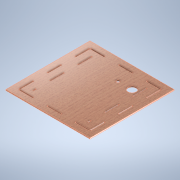
# Autodesk Inventor part: Roof_V2
Saved by Autodesk Inventor 2022.2 (Build 262287000, 287)
## iProperties
Created: 2022-11-15
Part Number: Roof_V2
Material: Generic
Document SubType Name: Modeling
Designer: jaege
Density: 1 g/cm^3
Appearance: Red Oak - Natural Low Gloss
Mass: 344.053 g
Surface Area: 1843.39 cm^2
Volume: 344.053 cm^3
Author: jaege
Autodesk Inventor part; units mm, degrees
ref_plane "YZ Plane" through (0, 0, 0) normal (1, 0, 0) x (0, 1, 0)
ref_plane "XZ Plane" through (0, 0, 0) normal (0, 1, 0) x (-1, 0, 0)
ref_plane "XY Plane" through (0, 0, 0) normal (0, 0, 1) x (1, 0, 0)
sketch "Sketch1" plane through (0, 0, 0) normal (0, 0, 1) x (1, 0, 0)
  line L0 (120, -66) -> (20, -66) construction
  line L1 (20, -66) -> (20, -26) construction
  line L2 (20, -26) -> (120, -26) construction
  line L3 (120, -26) -> (120, -66) construction
  line L4 (-275, -71) -> (125, -71) construction
  line L5 (125, -71) -> (125, 329) construction
  line L6 (125, 329) -> (-275, 329) construction
  line L7 (-275, 329) -> (-275, -71) construction
  line L8 (50, 104) -> (50, 154) construction
  line L9 (50, 154) -> (54, 154) construction
  line L10 (54, 154) -> (54, 104) construction
  line L11 (54, 104) -> (50, 104) construction
  line L12 (-50, 254) -> (-100, 254) construction
  line L13 (-100, 254) -> (-100, 258) construction
  line L14 (-100, 258) -> (-50, 258) construction
  line L15 (-50, 258) -> (-50, 254) construction
  line L16 (50, 258) -> (50, 254) construction
  line L17 (50, 254) -> (54, 254) construction
  line L18 (54, 254) -> (54, 204) construction
  line L19 (54, 204) -> (50, 204) construction
  line L20 (50, 204) -> (50, 254) construction
  line L21 (50, 254) -> (0, 254) construction
  line L22 (0, 254) -> (0, 258) construction
  line L23 (0, 258) -> (50, 258) construction
  line L24 (54, 4) -> (50, 4) construction
  line L25 (50, 4) -> (50, 0) construction
  line L26 (50, 0) -> (0, 0) construction
  line L27 (0, 0) -> (0, 4) construction
  line L28 (0, 4) -> (50, 4) construction
  line L29 (50, 4) -> (50, 54) construction
  line L30 (50, 54) -> (54, 54) construction
  line L31 (54, 54) -> (54, 4) construction
  line L32 (-100, 4) -> (-50, 4) construction
  line L33 (-50, 4) -> (-50, 0) construction
  line L34 (-50, 0) -> (-100, 0) construction
  line L35 (-100, 0) -> (-100, 4) construction
  line L36 (-204, 254) -> (-200, 254) construction
  line L37 (-200, 254) -> (-200, 258) construction
  line L38 (-200, 258) -> (-150, 258) construction
  line L39 (-150, 258) -> (-150, 254) construction
  line L40 (-150, 254) -> (-200, 254) construction
  line L41 (-200, 254) -> (-200, 204) construction
  line L42 (-200, 204) -> (-204, 204) construction
  line L43 (-204, 204) -> (-204, 254) construction
  line L44 (-200, 154) -> (-200, 104) construction
  line L45 (-200, 104) -> (-204, 104) construction
  line L46 (-204, 104) -> (-204, 154) construction
  line L47 (-204, 154) -> (-200, 154) construction
  line L48 (-200, 54) -> (-200, 4) construction
  line L49 (-200, 4) -> (-150, 4) construction
  line L50 (-150, 4) -> (-150, 0) construction
  line L51 (-150, 0) -> (-200, 0) construction
  line L52 (-200, 0) -> (-200, 4) construction
  line L53 (-200, 4) -> (-204, 4) construction
  line L54 (-204, 4) -> (-204, 54) construction
  line L55 (-204, 54) -> (-200, 54) construction
  line L56 (-275, -71) -> (125, -71) construction
  line L57 (125, -71) -> (125, 329) construction
  line L58 (125, 329) -> (-275, 329) construction
  line L59 (-275, 329) -> (-275, -71) construction
  line L60 (-275, -71) -> (125, 329) construction
  line L61 (75, 279) -> (-225, 279)
  line L62 (-225, 279) -> (-225, -21)
  line L63 (-225, -21) -> (75, -21)
  line L64 (75, -21) -> (75, 279)
  line L65 (75, 279) -> (-225, -21) construction
  line L66 (-225, 279) -> (75, -21) construction
  line L67 (-204, 4) -> (-200, 4)
  line L68 (-200, 4) -> (-200, 54)
  line L69 (-200, 54) -> (-204, 54)
  line L70 (-204, 54) -> (-204, 4)
  line L71 (-200, 104) -> (-204, 104)
  line L72 (-204, 104) -> (-204, 154)
  line L73 (-204, 154) -> (-200, 154)
  line L74 (-200, 154) -> (-200, 104)
  line L75 (-200, 204) -> (-204, 204)
  line L76 (-204, 204) -> (-204, 254)
  line L77 (-204, 254) -> (-200, 254)
  line L78 (-200, 254) -> (-200, 204)
  line L79 (-200, 254) -> (-150, 254)
  line L80 (-150, 254) -> (-150, 258)
  line L81 (-150, 258) -> (-200, 258)
  line L82 (-200, 258) -> (-200, 254)
  line L83 (-100, 254) -> (-50, 254)
  line L84 (-50, 254) -> (-50, 258)
  line L85 (-50, 258) -> (-100, 258)
  line L86 (-100, 258) -> (-100, 254)
  line L87 (0, 254) -> (50, 254)
  line L88 (50, 254) -> (50, 258)
  line L89 (50, 258) -> (0, 258)
  line L90 (0, 258) -> (0, 254)
  line L91 (50, 254) -> (54, 254)
  line L92 (54, 254) -> (54, 204)
  line L93 (54, 204) -> (50, 204)
  line L94 (50, 204) -> (50, 254)
  line L95 (54, 154) -> (50, 154)
  line L96 (50, 154) -> (50, 104)
  line L97 (50, 104) -> (54, 104)
  line L98 (54, 104) -> (54, 154)
  line L99 (54, 4) -> (50, 4)
  line L100 (50, 4) -> (50, 54)
  line L101 (50, 54) -> (54, 54)
  line L102 (54, 54) -> (54, 4)
  line L103 (50, 4) -> (0, 4)
  line L104 (0, 4) -> (0, 0)
  line L105 (0, 0) -> (50, 0)
  line L106 (50, 0) -> (50, 4)
  line L107 (-100, 0) -> (-50, 0)
  line L108 (-50, 0) -> (-50, 4)
  line L109 (-50, 4) -> (-100, 4)
  line L110 (-100, 4) -> (-100, 0)
  line L111 (-200, 0) -> (-150, 0)
  line L112 (-150, 0) -> (-150, 4)
  line L113 (-150, 4) -> (-200, 4)
  line L114 (-200, 4) -> (-200, 0)
  point P0 (-75, 129)
  dimension "d0" = 300
  dimension "d1" = 300
  constraints: 118 end point, 28 parallel, 14 horizontal, 14 perpendicular, 3 midpoint
  measures "d0" distance of L63.end L62.end
  measures "d1" distance of L62.end L61.end
extrude "Extrusion1" add sketch "Sketch1" against normal blind 4
sketch "Sketch2" plane through (0, 0, 0) normal (0, 0, 1) x (1, 0, 0)
  line L0 (-175, 234) -> (-171, 234)
  line L1 (-171, 234) -> (-171, 184)
  line L2 (-171, 184) -> (-175, 184)
  line L3 (-175, 184) -> (-175, 234)
  line L4 (-175, 184) -> (-171, 184)
  line L5 (-171, 184) -> (-171, 134)
  line L6 (-171, 134) -> (-175, 134)
  line L7 (-175, 134) -> (-175, 184)
  line L8 (-175, 134) -> (-171, 134)
  line L9 (-171, 134) -> (-171, 84)
  line L10 (-171, 84) -> (-175, 84)
  line L11 (-175, 84) -> (-175, 134)
  line L12 (-200, 254) -> (-200, 204) projected
  line L13 (-150, 254) -> (-200, 254) projected
  line L14 (-175, 84) -> (-171, 84)
  line L15 (-171, 84) -> (-171, 34)
  line L16 (-171, 34) -> (-175, 34)
  line L17 (-175, 34) -> (-175, 84)
  line L18 (-175, 34) -> (-171, 34)
  line L19 (-171, 34) -> (-171, 24)
  line L20 (-171, 24) -> (-175, 24)
  line L21 (-175, 24) -> (-175, 34)
  line L22 (-200, 4) -> (-150, 4) projected
  line L23 (25, 184) -> (21, 184)
  line L24 (21, 184) -> (25, 184)
  line L25 (21, 234) -> (25, 234)
  line L26 (25, 234) -> (25, 184)
  line L27 (21, 184) -> (21, 234)
  line L28 (25, 184) -> (25, 134)
  line L29 (25, 134) -> (21, 134)
  line L30 (21, 134) -> (25, 134)
  line L31 (25, 134) -> (25, 84)
  line L32 (25, 84) -> (21, 84)
  line L33 (21, 84) -> (21, 134)
  line L34 (21, 134) -> (21, 184)
  line L35 (21, 84) -> (25, 84)
  line L36 (25, 84) -> (25, 34)
  line L37 (21, 34) -> (21, 84)
  line L38 (25, 34) -> (21, 34)
  line L39 (21, 34) -> (25, 34)
  line L40 (25, 34) -> (25, 24)
  line L41 (21, 24) -> (21, 34)
  line L42 (25, 24) -> (21, 24)
  circle A0 centre (0, 204) radius 15
  line L43 (50, 254) -> (0, 254) projected
  line L44 (50, 204) -> (50, 254) projected
  point P0 (0, 0)
  point P1 (-173, 234)
  point P2 (-173, 24)
  point P3 (23, 234)
  point P4 (23, 24)
  point P5 (23, 234)
  point P6 (-75, 184)
  dimension "d4" = 4
  dimension "d5" = 50
  dimension "d6" = 4
  dimension "d7" = 50
  dimension "d8" = 4
  dimension "d9" = 50
  dimension "d10" = 25
  dimension "d11" = 20
  dimension "d12" = 4
  dimension "d13" = 50
  dimension "d14" = 4
  dimension "d15" = 20
  dimension "d20" = 196
  dimension "d25" = 30
  dimension "d29" = 50
  dimension "d30" = 50
  constraints: 80 end point, 10 parallel, 6 horizontal, 5 perpendicular, 3 midpoint, 1 centre point, 38 other
  measures "d4" distance of L1.end L2.end
  measures "d5" distance of L0.end L1.end
  measures "d6" distance of L5.end L6.end
  measures "d7" distance of L4.end L5.end
  measures "d8" distance of L9.end L10.end
  measures "d9" distance of L8.end L9.end
  measures "d10" distance from line of L12 L0.start
  measures "d11" distance from line of L13 point (-173, 234)
  measures "d12" distance of L15.end L16.end
  measures "d13" distance of L14.end L15.end
  measures "d14" distance of L19.end L20.end
  measures "d15" distance from line of L22 point (-173, 24)
  measures "d20" distance of L2.end L23.end
  measures "d25" diameter of A0
  measures "d29" distance of L43.end A0.centre
  measures "d30" distance from line of L44 A0.centre
extrude "Extrusion2" cut sketch "Sketch2" against normal blind 10 contours L0 L1 L2 L3 | L6 L9 L10 L11 | L16 L19 L20 L21 | L23 L27 L25 L26 | L31 L32 L33 L29 | L40 L42 L41 L38 | A0
sketch "Sketch3" plane through (0, 0, 0) normal (0, 0, 1) x (1, 0, 0)
  circle A0 centre (-50, 204) radius 6
  line L0 (-50, 254) -> (-100, 254) projected
  circle A1 centre (0, 204) radius 15 projected
  point P0 (0, 0)
  dimension "d31" = 12
  dimension "d32" = 50
  dimension "d33" = 50
  constraints: 1 centre point
  measures "d31" diameter of A0
  measures "d32" distance from line of A0.centre L0
  measures "d33" distance of A1.centre A0.centre
extrude "Extrusion3" cut sketch "Sketch3" against normal through all contours A0
body "Solid1"
